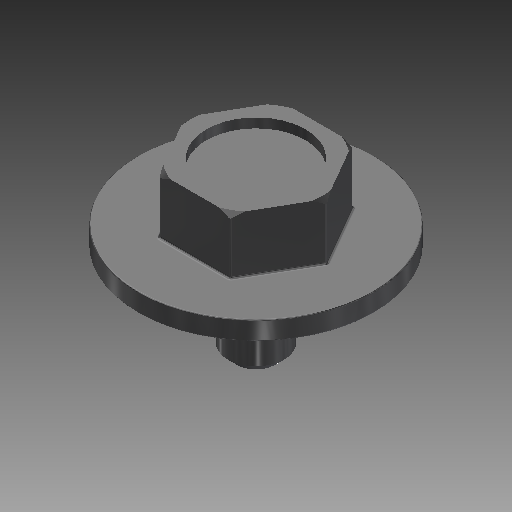
# Autodesk Inventor part: 318-04
Saved by Autodesk Inventor 2019 (Build 230136000, 136)
## iProperties
Company: Autodesk Inc.
Created: 2007-10-26
Part Number: 318-04
Document SubType Name: Modeling
Designer: Autodesk Inc.
Density: 8 g/cm^3
Mass: 16.3773 g
Surface Area: 16.0193 cm^2
Volume: 2.04717 cm^3
Material: Stainless Steel
Description: SCREW
Appearance: Rubber - Black - Version 1.1
Component Category: Fasteners
Author: Inventor
Autodesk Inventor part; units mm, degrees
ref_plane "YZ Plane" through (0, 0, 0) normal (1, 0, 0) x (0, 1, 0)
sketch "Sketch1" plane through (0, 0, 0) normal (0, 0, 1) x (1, 0, 0)
  line L0 (0, -13.4) -> (0, 10.4) projected
  line L1 (-2.5052, 0) -> (15.0311, 0) projected
  line L2 (0, 7) -> (5.25, 7)
  line L3 (5.25, 7) -> (5.25, 2)
  line L4 (5.25, 2) -> (12.375, 2)
  line L5 (12.5, 1.875) -> (12.5, 0.125)
  line L6 (12.375, 0) -> (3, 0)
  line L7 (3, 0) -> (3, -9)
  line L8 (3, -9) -> (2, -10)
  line L9 (2, -10) -> (0, -10)
  arc A0 (12.5, 1.875) -> (12.375, 2) centre (12.375, 1.875) ccw
  arc A1 (12.375, 0) -> (12.5, 0.125) centre (12.375, 0.125) ccw
  point P0 (0, 0)
  point P1 (12.5, 2)
  point P2 (12.5, 0)
  dimension "d0" = 1
  dimension "d1" = 1
  dimension "d2" = 6
  dimension "d3" = 25
  dimension "d4" = 10.5
  dimension "d5" = 2
  dimension "d7" = 10
  dimension "d10" = 5
  dimension "d12" = 0.125
  constraints: 16 end point, 6 point on line, 5 parallel, 4 point on circle, 4 tangent, 2 centre point, 2 perpendicular, 1 collinear, 1 equal radius
  measures "d0" horizontal distance of L7.end L8.end
  measures "d1" horizontal distance of L7.end L8.end
  measures "d2" diameter of L7 L0
  measures "d3" diameter of L5 L0
  measures "d4" diameter of L3 L0
  measures "d5" distance between parallel lines of L4 L6
  measures "d7" distance between parallel lines of L9 L6
  measures "d10" distance between parallel lines of L4 L2
  measures "d12" radius of A0
revolve "Revolution1" add sketch "Sketch1" angle 360 about axis through (0, -10, 0) along (0, 1, 0)
ref_plane "Work Plane1" through (0, 8, 0) normal (0, 1, 0) x (-1, 0, 0)
sketch "Sketch2" plane through (0, 8, 0) normal (0, 1, 0) x (-1, 0, 0)
  line L0 (10.5078, 0) -> (-10.5078, 0) projected
  line L1 (0, -9.1) -> (0, 9.1) projected
  line L2 (-3.7528, -6.5) -> (-7.5056, 0)
  line L3 (-7.5056, 0) -> (-3.7528, 6.5)
  line L4 (-3.7528, 6.5) -> (3.7528, 6.5)
  line L5 (3.7528, 6.5) -> (7.5056, 0)
  line L6 (7.5056, 0) -> (3.7528, -6.5)
  line L7 (3.7528, -6.5) -> (-3.7528, -6.5)
  circle A0 centre (0, 0) radius 5.25
  dimension "d16" = 13
  dimension "d17" = 10.5
  constraints: 12 end point, 2 coincident, 1 centre point, 1 parallel, 13 other
  measures "d16" distance between parallel lines of L4 L7
  measures "d17" diameter of A0
extrude "Extrusion1" add sketch "Sketch2" against normal up to surface (6 mm away) contours L6 L7 L1 A0 L0 | L0 A0 L1 L4 L5 | A0 L0 L3 L4 L1 | L1 L7 L2 L0 A0
fillet "Fillet1" radius 0.25 12 edges at (-5.6292, 2, 3.25) (-5.6292, 2, -3.25) (0, 2, 6.5) (5.6292, 2, 3.25) (5.6292, 2, -3.25) (0, 2, -6.5) (3.7528, 5, -6.5) (7.5056, 5, 0) (3.7528, 5, 6.5) (-3.7528, 5, -6.5) (-3.7528, 5, 6.5) (-7.5056, 5, 0)
ref_plane "Work Plane2" through (0, 0, 0) normal (0, 0, 1) x (1, 0, 0)
sketch "Sketch3" plane through (0, 0, 0) normal (0, 0, 1) x (1, 0, 0)
  line L0 (-7.5, 7.5) -> (-7.5, 8)
  line L1 (-7.5, 8) -> (-7, 8)
  line L2 (0, -1.6) -> (0, 9.6) projected
  line L3 (-9, 0) -> (1.5, 0) projected
  line L4 (-7, 8) -> (-7.5, 7.5)
  point P0 (0, 0)
  dimension "d22" = 0.5
  dimension "d23" = 0.5
  dimension "d26" = 7.5
  dimension "d27" = 8
  constraints: 6 end point, 1 perpendicular
  measures "d22" distance of L0.end L1.end
  measures "d23" distance of L0.start L0.end
  measures "d26" distance between parallel lines of L0 L2
  measures "d27" distance between parallel lines of L3 L1
revolve "Revolution2" cut sketch "Sketch3" angle 360 about axis through (0, -10, 0) along (0, 1, 0)
body "Solid1"
